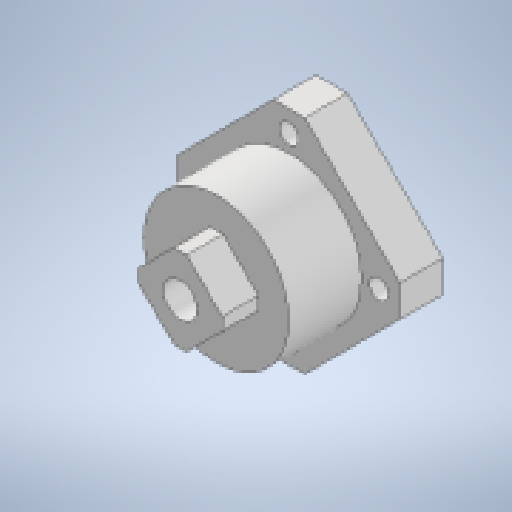
# Autodesk Inventor part: FK10
Saved by Autodesk Inventor 2023 (Build 270158000, 158)
## iProperties
Created: 2022-04-30
Part Number: FK10
Material: Generic
Document SubType Name: Modeling
Designer: plebbb
Density: 1 g/cm^3
Appearance: Default
Author: plebbb
Autodesk Inventor part; units mm, degrees
ref_plane "YZ Plane" through (0, 0, 0) normal (1, 0, 0) x (0, 1, 0)
ref_plane "XZ Plane" through (0, 0, 0) normal (0, 1, 0) x (-1, 0, 0)
ref_plane "XY Plane" through (0, 0, 0) normal (0, 0, 1) x (1, 0, 0)
sketch "Sketch1" plane through (0, 0, 0) normal (0, 0, 1) x (1, 0, 0)
  line L0 (-26, -3.6985) -> (-3.6985, -26)
  line L1 (-3.6985, -26) -> (3.6985, -26)
  line L2 (3.6985, -26) -> (26, -3.6985)
  line L3 (26, -3.6985) -> (26, 3.6985)
  line L4 (26, 3.6985) -> (3.6985, 26)
  line L5 (3.6985, 26) -> (-3.6985, 26)
  line L6 (-3.6985, 26) -> (-26, 3.6985)
  line L7 (-26, 3.6985) -> (-26, -3.6985)
  circle A0 centre (0, 0) radius 5
  line L8 (-21, 0) -> (0, -21) construction
  line L9 (0, -21) -> (21, 0) construction
  line L10 (21, 0) -> (0, 21) construction
  line L11 (0, 21) -> (-21, 0) construction
  circle A1 centre (0, 21) radius 2.25
  circle A2 centre (-21, 0) radius 2.25
  circle A3 centre (0, -21) radius 2.25
  circle A4 centre (21, 0) radius 2.25
  point P0 (0, 26)
  point P1 (26, 0)
  dimension "d0" = 10
  dimension "d1" = 42
  dimension "d2" = 135
  dimension "d3" = 42
  dimension "d4" = 4.5
  dimension "d5" = 52
  constraints: 24 end point, 5 centre point, 5 coincident, 5 equal length, 5 horizontal alignment, 5 perpendicular, 5 vertical alignment, 3 equal radius, 2 midpoint, 2 vertical, 1 parallel
  measures "d0" diameter of A0
  measures "d1" distance between parallel lines of L4 L0
  measures "d2" angle of L7 L6
  measures "d3" distance of L8.end L10.end
  measures "d4" diameter of A1
  measures "d5" distance between parallel lines of L1 L5
extrude "Extrusion1" add sketch "Sketch1" along normal blind 10
sketch "Sketch2" plane through (0, 0, 10) normal (0, 0, 1) x (1, 0, 0)
  circle A0 centre (0, 0) radius 5 projected
  circle A1 centre (0, 0) radius 17
  dimension "d8" = 34
  constraints: 1 centre point, 1 coincident
  measures "d8" diameter of A1
extrude "Extrusion2" add sketch "Sketch2" along normal blind 17
sketch "Sketch3" plane through (0, 0, 0) normal (0, 0, -1) x (-1, 0, 0)
  circle A0 centre (0, 21) radius 4
  circle A1 centre (21, 0) radius 4
  circle A2 centre (0, -21) radius 4
  circle A3 centre (-21, 0) radius 4
  circle A4 centre (0, 21) radius 2.25 projected
  circle A5 centre (-21, 0) radius 2.25 projected
  circle A6 centre (21, 0) radius 2.25 projected
  circle A7 centre (0, -21) radius 2.25 projected
  point P0 (0, 0)
  dimension "d11" = 8
  constraints: 4 centre point, 4 concentric, 3 equal radius
  measures "d11" diameter of A0
extrude "Extrusion3" cut sketch "Sketch3" against normal blind 4 contours A0 | A1 | A2 | A3 | A4 | A5 | A6 | A7
sketch "Sketch5" plane through (0, 0, 27) normal (0, 0, 1) x (1, 0, 0)
  line L0 (-9.8137, 1.5) -> (-1.5, 9.8137)
  line L1 (-1.5, 9.8137) -> (1.5, 9.8137)
  line L2 (1.5, 9.8137) -> (9.8137, 1.5)
  line L3 (9.8137, 1.5) -> (9.8137, -1.5)
  line L4 (9.8137, -1.5) -> (1.5, -9.8137)
  line L5 (1.5, -9.8137) -> (-1.5, -9.8137)
  line L6 (-1.5, -9.8137) -> (-9.8137, -1.5)
  line L7 (-9.8137, -1.5) -> (-9.8137, 1.5)
  circle A0 centre (0, 0) radius 5
  point P0 (9.8137, 0)
  point P1 (-9.8137, 0)
  point P2 (0, 9.8137)
  point P3 (0, -9.8137)
  dimension "d14" = 16
  dimension "d15" = 3
  dimension "d16" = 10
  constraints: 16 end point, 4 midpoint, 3 equal length, 3 parallel, 2 horizontal, 2 horizontal alignment, 2 perpendicular, 2 vertical alignment, 1 centre point, 1 coincident
  measures "d14" distance between parallel lines of L4 L0
  measures "d15" distance of L0.end L1.end
  measures "d16" diameter of A0
extrude "Extrusion4" add sketch "Sketch5" along normal blind 8.5
body "Solid1"
